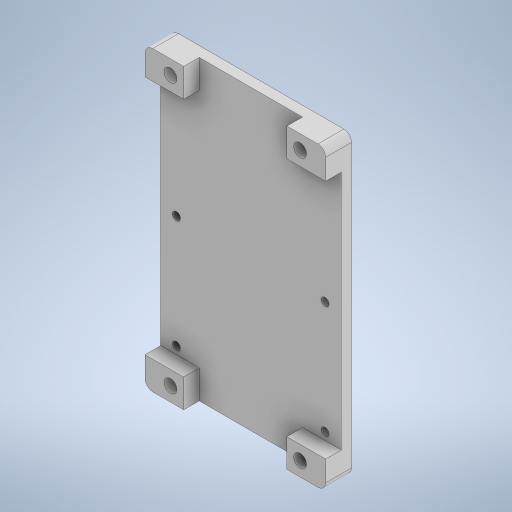
# Autodesk Inventor part: 와이파이 모듈 커버
Saved by Autodesk Inventor 2023 (Build 270158000, 158)
## iProperties
Created: 2022-06-24
Part Number: 와이파이 모듈 커버
Material: 일반
Document SubType Name: Modeling
Designer: user
Density: 1 g/cm^3
Appearance: 기본값
Author: user
Autodesk Inventor part; units mm, degrees
ref_plane "YZ Plane" through (0, 0, 0) normal (1, 0, 0) x (0, 1, 0)
ref_plane "XZ Plane" through (0, 0, 0) normal (0, 1, 0) x (-1, 0, 0)
ref_plane "XY Plane" through (0, 0, 0) normal (0, 0, 1) x (1, 0, 0)
sketch "스케치1" plane through (0, 0, 0) normal (0, 0, 1) x (1, 0, 0)
  line L0 (-16, 28.8) -> (16, 28.8)
  line L1 (17.5, 27.3) -> (17.5, -27.3)
  line L2 (16, -28.8) -> (-16, -28.8)
  line L3 (-17.5, -27.3) -> (-17.5, 27.3)
  line L4 (-17.5, 28.8) -> (17.5, -28.8) construction
  line L5 (17.5, 28.8) -> (-17.5, -28.8) construction
  circle A0 centre (-12.55, 26.05) radius 1.25
  line L6 (0, 0) -> (0, 21.4248) construction
  line L7 (0, 0) -> (10.8427, 0) construction
  circle A1 centre (12.55, 26.05) radius 1.25
  circle A2 centre (-12.55, -26.05) radius 1.25
  circle A3 centre (12.55, -26.05) radius 1.25
  arc A4 (-16, 28.8) -> (-17.5, 27.3) centre (-16, 27.3) ccw
  arc A5 (17.5, 27.3) -> (16, 28.8) centre (16, 27.3) ccw
  arc A6 (16, -28.8) -> (17.5, -27.3) centre (16, -27.3) ccw
  arc A7 (-17.5, -27.3) -> (-16, -28.8) centre (-16, -27.3) ccw
  line L8 (-17.5, 23.3) -> (17.5, 23.3)
  line L9 (-17.5, -23.3) -> (17.5, -23.3)
  line L10 (-10, 28.8) -> (10, 28.8)
  line L11 (10, 28.8) -> (10, 23.3)
  line L12 (10, 23.3) -> (-10, 23.3)
  line L13 (-10, 23.3) -> (-10, 28.8)
  line L14 (-10, 28.8) -> (10, 23.3) construction
  line L15 (10, 28.8) -> (-10, 23.3) construction
  line L16 (10, -28.8) -> (10, -23.3)
  line L17 (-10, -23.3) -> (-10, -28.8)
  point P0 (0, 26.05)
  point P1 (10, 26.05)
  point P2 (10, 28.8)
  dimension "d0" = 35
  dimension "d1" = 57.6
  dimension "d2" = 25.1
  dimension "d3" = 52.1
  dimension "d4" = 2.5
  dimension "d5" = 1.5
  dimension "d6" = 5.5
  dimension "d7" = 5.5
  dimension "d8" = 20
  constraints: 36 end point, 13 point on line, 8 centre point, 8 point on circle, 8 tangent, 7 symmetric about line, 5 midpoint, 4 parallel, 4 perpendicular, 3 equal radius, 3 horizontal, 1 vertical, 1 vertical alignment, 3 other
  measures "d0" distance of L4.end L5.end
  measures "d1" distance of L5.start L4.end
  measures "d2" distance of A1.centre A0.centre
  measures "d3" distance of A2.centre A0.centre
  measures "d4" diameter of A0
  measures "d5" radius of A4
  measures "d6" distance between parallel lines of L0 L8
  measures "d7" distance between parallel lines of L2 L9
  measures "d8" distance from line of point (10, 26.05) L13
extrude "돌출1" add sketch "스케치1" along normal blind 3 contours L0 L13 L8 L3 A4 | L0 A5 L1 L8 L11 | L9 L17 L2 A7 L3 | L1 A6 L2 L16 L9
extrude "돌출2" add sketch "스케치1" against normal blind 2
sketch "스케치3" plane through (0, 0, -2) normal (0, 0, -1) x (-1, 0, 0)
  line L0 (14.4, 0) -> (-14.4, 0)
  line L1 (-14.4, 0) -> (-14.4, -21.8)
  line L2 (-14.4, -21.8) -> (14.4, -21.8)
  line L3 (14.4, -21.8) -> (14.4, 0)
  line L4 (14.4, 0) -> (-14.4, -21.8) construction
  line L5 (-14.4, 0) -> (14.4, -21.8) construction
  point P0 (0, 0)
  point P1 (0, -10.9)
  point P2 (0, 0)
  dimension "d13" = 21.8
  dimension "d14" = 28.8
  constraints: 12 end point, 3 midpoint, 2 parallel, 1 coincident, 1 horizontal, 1 perpendicular, 1 vertical alignment
  measures "d13" distance of L2.end L0.start
  measures "d14" distance of L1.end L2.end
hole "구멍1" at (-14.4, 0, -2) at (14.4, 0, -2) at (14.4, -21.8, -2) at (-14.4, -21.8, -2) direction (0, 0, 1) diameter 1.567 end through all countersink diameter 3 countersink angle 90 thread size "M2x0.4" class "6H" standard "ISO Metric profile"
sketch "스케치4" plane through (0, 0, -2) normal (0, 0, -1) x (-1, 0, 0)
  circle A0 centre (12.55, -26.05) radius 1.25 projected
  circle A1 centre (12.55, -26.05) radius 1.75
  circle A2 centre (-12.55, -26.05) radius 1.25 projected
  circle A3 centre (-12.55, -26.05) radius 1.75
  circle A4 centre (12.55, 26.05) radius 1.25 projected
  circle A5 centre (12.55, 26.05) radius 1.75
  circle A6 centre (-12.55, 26.05) radius 1.75
  point P0 (0, 0)
  dimension "d22" = 3.5
  dimension "d23" = 3.5
  dimension "d24" = 3.5
  dimension "d25" = 3.5
  constraints: 4 centre point, 3 coincident
  measures "d22" diameter of A1
  measures "d23" diameter of A3
  measures "d24" diameter of A5
  measures "d25" diameter of A6
extrude "돌출3" cut sketch "스케치4" against normal blind 2 contours A0 | A1 | A2 | A3 | A4 | A5 | A6
sketch "스케치5" plane through (0, 0, -2) normal (0, 0, -1) x (-1, 0, 0)
  line L0 (13.97, 4.25) -> (-13.97, 4.25)
  line L1 (-13.97, 4.25) -> (-13.97, 21.75)
  line L2 (-13.97, 21.75) -> (13.97, 21.75)
  line L3 (13.97, 21.75) -> (13.97, 4.25)
  line L4 (13.97, 4.25) -> (-13.97, 21.75) construction
  line L5 (-13.97, 4.25) -> (13.97, 21.75) construction
  line L6 (13.97, 2.5) -> (-13.97, 2.5)
  line L7 (-13.97, 2.5) -> (-13.97, 23.5)
  line L8 (-13.97, 23.5) -> (13.97, 23.5)
  line L9 (13.97, 23.5) -> (13.97, 2.5)
  line L10 (13.97, 2.5) -> (-13.97, 23.5) construction
  line L11 (-13.97, 2.5) -> (13.97, 23.5) construction
  point P0 (0, 0)
  point P1 (0, 13)
  point P2 (13.97, 4.25)
  point P3 (-13.97, 4.25)
  dimension "d28" = 27.94
  dimension "d29" = 17.5
  dimension "d30" = 21
  dimension "d31" = 13
  constraints: 24 end point, 4 midpoint, 4 parallel, 2 horizontal, 2 perpendicular, 1 vertical alignment
  measures "d28" distance of L0.start L0.end
  measures "d29" distance of L0.end L1.end
  measures "d30" distance between parallel lines of L8 L6
  measures "d31" distance of point (0, 0) point (0, 13)
extrude "돌출4" add sketch "스케치5" along normal blind 3 contours L9 L6 L7 L0 | L2 L7 L8 L9
